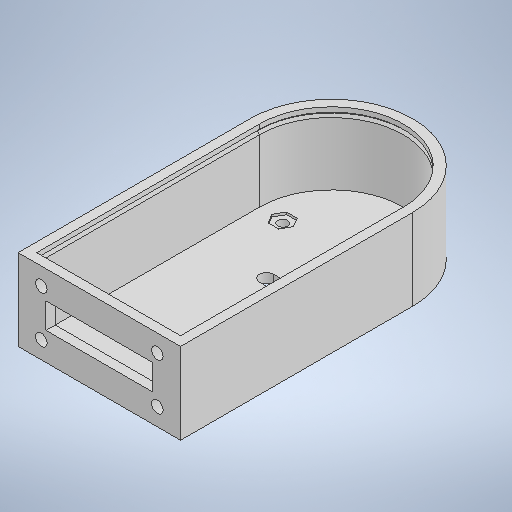
# Autodesk Inventor part: SCARA arm
Saved by Autodesk Inventor 2025.2 (Build 292293000, 293)
## iProperties
Created: 2025-01-27
Part Number: SCARA arm
Material: Generic
Document SubType Name: Modeling
Designer: caomi
Density: 1 g/cm^3
Appearance: Default
Author: caomi
Autodesk Inventor part; units mm, degrees
ref_plane "YZ Plane" through (0, 0, 0) normal (1, 0, 0) x (0, 1, 0)
ref_plane "XZ Plane" through (0, 0, 0) normal (0, 1, 0) x (-1, 0, 0)
ref_plane "XY Plane" through (0, 0, 0) normal (0, 0, 1) x (1, 0, 0)
sketch "Sketch1" plane through (0, 0, 0) normal (0, 1, 0) x (-1, 0, 0)
  line L0 (0, 0) -> (70, 0)
  line L1 (70, 0) -> (70, -100)
  line L2 (70, -100) -> (0, -100)
  line L3 (0, -100) -> (0, 0)
  circle A0 centre (35, -100) radius 35
  point P0 (0, -100)
  dimension "d0" = 70
  dimension "d1" = 100
  constraints: 8 end point, 2 parallel, 1 horizontal, 1 midpoint, 1 perpendicular, 3 other
  measures "d0" distance of L0.start L0.end
  measures "d1" distance between parallel lines of L2 L0
extrude "Extrusion1" add sketch "Sketch1" along normal blind 35
shell "Shell1" thickness 4 removed faces 1 at (-23.3333, 35, -33.3333)
sketch "Sketch2" plane through (-70, 0, 0) normal (0, 0, 1) x (1, 0, 0)
  line L0 (35, 44.7542) -> (35, -30.4775) construction
  line L1 (75.874, 17.5) -> (-5.874, 17.5) construction
  line L2 (0, 35) -> (70, 35) projected
  line L3 (70, 0) -> (70, 35) projected
  line L4 (0, 0) -> (0, 35) projected
  line L5 (0, 0) -> (70, 0) projected
  line L6 (58, 23) -> (12, 23)
  line L7 (12, 23) -> (12, 12)
  line L8 (12, 12) -> (58, 12)
  line L9 (58, 12) -> (58, 23)
  circle A0 centre (10, 27.5) radius 2.5
  circle A1 centre (60, 7.5) radius 2.5
  circle A2 centre (10, 7.5) radius 2.5
  circle A3 centre (60, 27.5) radius 2.5
  point P0 (35, 17.5)
  point P1 (35, 35)
  point P2 (70, 17.5)
  dimension "d7" = 12
  dimension "d8" = 5
  dimension "d9" = 50
  dimension "d10" = 20
  constraints: 12 end point, 4 centre point, 3 midpoint, 3 point on line, 1 equal radius, 1 horizontal, 1 symmetric about line, 1 vertical, 5 other
  measures "d7" distance between parallel lines of L2 L6
  measures "d8" diameter of A1
  measures "d9" distance of A1.centre A2.centre
  measures "d10" distance of A3.centre A1.centre
extrude "Extrusion2" cut sketch "Sketch2" against normal blind 50 contours L9 L8 L7 L6 | A0 | A1 | A2 | A3
ref_plane "Work Plane2" through (0, 32, 0) normal (0, 1, 0) x (1, 0, 0)
sketch "Sketch4" plane through (0, 32, 0) normal (0, 1, 0) x (1, 0, 0)
  line L0 (-66, 4) -> (-66, 100) projected
  arc A0 (-4, 100) -> (-66, 100) centre (-35, 100) ccw projected
  line L1 (-4, 100) -> (-4, 4) projected
  line L2 (-4, 4) -> (-66, 4) projected
  point P0 (0, 0)
ref_plane "Work Plane3" through (-66, 32, -4) normal (0, 0, -1) x (-1, 0, 0)
sketch "Sketch5" plane through (-66, 32, -4) normal (0, 0, -1) x (-1, 0, 0)
  line L0 (0, 1) -> (1, 0)
  line L1 (1, 0) -> (0, -1)
  line L2 (0, -1) -> (0, 1)
  line L3 (2.655, 0) -> (0.8949, 0) construction
  point P0 (-66, -32)
  point P1 (0, 0)
  point P2 (0, 0)
  point P3 (0, 0)
  dimension "d29" = 1
  dimension "d30" = 45
  constraints: 8 end point, 1 horizontal, 1 horizontal alignment, 1 midpoint, 1 point on line, 1 vertical, 1 other
  measures "d29" distance from line of L2 L0.end
  measures "d30" angle of L0 L3
sweep "Sweep1" cut profiles "Sketch5" path "Sketch4"
sketch "Sketch6" plane through (-35, 4, -100) normal (0, 1, 0) x (1, 0, 0)
  circle A0 centre (-21, 0) radius 2.15
  circle A1 centre (21, 0) radius 2.15
  line L0 (0, -2.8251) -> (0, 10.2985) construction
  arc A2 (31, 0) -> (-31, 0) centre (0, 0) ccw projected
  line L1 (3, -25) -> (-3, -25) construction
  line L2 (3, -22) -> (-3, -22)
  line L3 (-3, -28) -> (3, -28)
  arc A3 (3, -28) -> (3, -22) centre (3, -25) ccw
  arc A4 (-3, -22) -> (-3, -28) centre (-3, -25) ccw
  point P0 (35, -100)
  point P1 (0, 31)
  point P2 (0, -25)
  dimension "d33" = 4.3
  dimension "d34" = 42
  dimension "d37" = 6
  dimension "d38" = 6
  dimension "d39" = 25
  constraints: 10 end point, 5 point on circle, 4 centre point, 4 tangent, 2 point on line, 1 horizontal alignment, 1 midpoint, 1 parallel, 1 perpendicular, 1 vertical, 1 other
  measures "d33" diameter of A1
  measures "d34" distance of A1.centre A0.centre
  measures "d37" distance between parallel lines of L2 L3
  measures "d38" distance of L3.start L3.end
  measures "d39" distance from line of A2.centre L1
extrude "Extrusion5" cut sketch "Sketch6" against normal blind 50
sketch "Sketch7" plane through (-35, 4, -100) normal (0, 1, 0) x (1, 0, 0)
  line L0 (-23.3094, 4) -> (-18.6906, 4)
  line L1 (-18.6906, 4) -> (-16.3812, 0)
  line L2 (-16.3812, 0) -> (-18.6906, -4)
  line L3 (-18.6906, -4) -> (-23.3094, -4)
  line L4 (-23.3094, -4) -> (-25.6188, 0)
  line L5 (-25.6188, 0) -> (-23.3094, 4)
  circle A0 centre (-21, 0) radius 2.15 projected
  circle A1 centre (21, 0) radius 2.15 projected
  line L6 (23.3094, 4) -> (25.6188, 0)
  line L7 (25.6188, 0) -> (23.3094, -4)
  line L8 (23.3094, -4) -> (18.6906, -4)
  line L9 (18.6906, -4) -> (16.3812, 0)
  line L10 (16.3812, 0) -> (18.6906, 4)
  line L11 (18.6906, 4) -> (23.3094, 4)
  point P0 (35, -100)
  point P1 (-21, -4)
  dimension "d40" = 8
  constraints: 24 end point, 2 coincident, 2 horizontal, 1 collinear, 1 midpoint, 26 other
  measures "d40" distance from line of point (-21, -4) L0
extrude "Extrusion6" cut sketch "Sketch7" against normal blind 1
equation "\"d11\" = d9"
equation "\"d35\" = d9"
body "Solid1"
